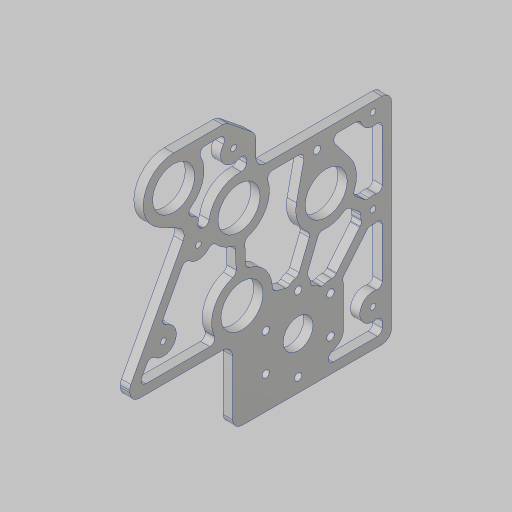
# Autodesk Inventor part: CL4-016
Saved by Autodesk Inventor 2023.5 (Build 275446000, 446)
## iProperties
Created: 2025-02-08
Part Number: CL4-016
Material: Aluminum 6061
Document SubType Name: Modeling
Designer: slick
Density: 2.7 g/cm^3
Appearance: Aluminum - Flat
Author: slick
Autodesk Inventor part; units mm, degrees
ref_plane "YZ Plane" through (0, 0, 0) normal (1, 0, 0) x (0, 1, 0)
ref_plane "XZ Plane" through (0, 0, 0) normal (0, 1, 0) x (-1, 0, 0)
ref_plane "XY Plane" through (0, 0, 0) normal (0, 0, 1) x (1, 0, 0)
sketch "Sketch1" plane through (0, 0, 0) normal (1, 0, 0) x (0, 1, 0)
  line L0 (0, 0) -> (304.8, 0) construction
  line L1 (304.8, 0) -> (304.8, 25.4) construction
  line L2 (304.8, 25.4) -> (0, 25.4) construction
  line L3 (0, 25.4) -> (0, 0) construction
  line L4 (304.8053, 47.8215) -> (292.8807, 25.3947) construction
  line L5 (292.8807, 25.3947) -> (44.6826, 157.364) construction
  line L6 (44.6826, 157.364) -> (56.6072, 179.7908) construction
  line L7 (56.6072, 179.7908) -> (304.8053, 47.8215) construction
  line L8 (50.8, 179.7908) -> (0, 179.7908) construction
  line L9 (0, 179.7908) -> (0, 154.3908) construction
  line L10 (0, 154.3908) -> (50.8, 154.3908) construction
  line L11 (50.8, 154.3908) -> (50.8, 179.7908) construction
  circle A0 centre (320.675, 23.9014) radius 45.3644 construction
  line L12 (0, 0) -> (50.8, 0) construction
  line L13 (50.8, 0) -> (50.8, -25.4) construction
  line L14 (50.8, -25.4) -> (0, -25.4) construction
  line L15 (0, -25.4) -> (0, 0) construction
  line L16 (50.8, -25.4) -> (558.8, -25.4) construction
  point P0 (292.1, 12.7)
  point P1 (304.8, 12.7)
  point P2 (287.6296, 42.5704)
  point P3 (298.843, 36.6081)
  point P4 (0, 167.0908)
  point P5 (0, 12.7)
  dimension "d0" = 25.4
  dimension "d1" = 304.8
  dimension "d2" = 28
  dimension "d3" = 12.7
  dimension "d4" = 12.7
  dimension "d5" = 12.7
  dimension "d6" = 25.4
  dimension "d7" = 281.1018
  dimension "d8" = 4.4704
  dimension "d9" = 29.8704
  dimension "d10" = 50.8
  dimension "d11" = 25.4
  dimension "d12" = 50.8
  dimension "d13" = 25.4
  dimension "d14" = 508
  dimension "d15" = 90.7288
  dimension "d16" = 28.575
  dimension "d17" = 11.2014
  constraints: 34 end point, 8 parallel, 4 horizontal, 4 midpoint, 4 perpendicular, 2 horizontal alignment, 1 centre point, 1 vertical alignment
  measures "d0" distance of L1.end L0.end
  measures "d1" distance of L0.start L0.end
  measures "d2" angle of L2 L5
  measures "d3" distance of point (292.1, 12.7) point (304.8, 12.7)
  measures "d4" distance of point (287.63, 42.57) point (298.843, 36.608)
  measures "d5" distance from line of L7 point (287.63, 42.57)
  measures "d6" distance of L4.start L4.end
  measures "d7" distance of L6.end L4.start
  measures "d8" horizontal distance of point (292.1, 12.7) point (287.63, 42.57)
  measures "d9" vertical distance of point (292.1, 12.7) point (287.63, 42.57)
  measures "d10" distance of L10.end L9.end
  measures "d11" distance of L9.end L8.end
  measures "d12" distance of L13.end L14.end
  measures "d13" distance of L12.end L13.end
  measures "d14" distance of L13.end L16.end
  measures "d15" diameter of A0
  measures "d16" horizontal distance of point (292.1, 12.7) A0.centre
  measures "d17" vertical distance of point (292.1, 12.7) A0.centre
sketch "Sketch2" plane through (0, 0, 0) normal (1, 0, 0) x (0, 1, 0)
  circle A0 centre (320.675, 23.9014) radius 45.3644 construction
  line L0 (50.8, -25.4) -> (558.8, -25.4) construction
  line L1 (50.8, 0) -> (50.8, -25.4) construction
  line L2 (0, 0) -> (50.8, 0) construction
  line L3 (50.8, -25.4) -> (0, -25.4) construction
  line L4 (0, -25.4) -> (0, 0) construction
  line L5 (0, 25.4) -> (0, 0) construction
  line L6 (304.8053, 47.8215) -> (292.8807, 25.3947) construction
  line L7 (304.8, 0) -> (304.8, 25.4) construction
  line L8 (56.6072, 179.7908) -> (304.8053, 47.8215) construction
  line L9 (50.8, 154.3908) -> (50.8, 179.7908) construction
  line L10 (44.6826, 157.364) -> (56.6072, 179.7908) construction
  line L11 (0, 0) -> (304.8, 0) construction
  line L12 (304.8, 25.4) -> (0, 25.4) construction
  line L13 (0, 154.3908) -> (50.8, 154.3908) construction
  line L14 (50.8, 179.7908) -> (0, 179.7908) construction
  line L15 (292.8807, 25.3947) -> (44.6826, 157.364) construction
  line L16 (0, 179.7908) -> (0, 154.3908) construction
  circle A1 centre (34.925, 63.5) radius 30.48 construction
  circle A2 centre (34.925, 63.5) radius 6.35 construction
  circle A3 centre (70.4169, 101.6) radius 45.72 construction
  circle A4 centre (70.4169, 101.6) radius 12.7 construction
  circle A5 centre (128.803, 103.5908) radius 45.72 construction
  circle A6 centre (128.803, 103.5908) radius 12.7 construction
  circle A7 centre (162.718, 148.0019) radius 43.18 construction
  arc A8 (285.6013, 0) -> (341.9337, 60.6371) centre (320.675, 23.9014) ccw construction
  arc A9 (169.8042, 160.2472) -> (152.4976, 138.2191) centre (162.718, 148.0019) ccw construction
  line L17 (169.8042, 160.2472) -> (341.9337, 60.6371) construction
  line L18 (290.0139, -5.4472) -> (152.4976, 138.2191) construction
  circle A10 centre (128.803, 103.5908) radius 14.2875
  circle A11 centre (162.718, 148.0019) radius 14.2875
  circle A12 centre (70.4169, 101.6) radius 14.2875
  circle A13 centre (34.925, 63.5) radius 14.2875 construction
  circle A14 centre (128.803, 103.5908) radius 20.6375 construction
  circle A15 centre (162.718, 148.0019) radius 20.6375 construction
  circle A16 centre (70.4169, 101.6) radius 20.6375 construction
  circle A17 centre (34.925, 63.5) radius 20.6375 construction
  line L19 (185.2061, 97.0299) -> (95.4986, 144.7283) construction
  line L20 (165.1, 12.7) -> (25.4, 12.7) construction
  line L21 (0, 0) -> (190.5, 0)
  line L22 (190.5, 0) -> (190.5, 177.8)
  line L23 (190.5, 177.8) -> (0, 177.8)
  line L24 (0, 177.8) -> (0, 0)
  circle A18 centre (34.925, 63.5) radius 10.16
  circle A19 centre (34.925, 63.5) radius 25.4 construction
  point P0 (0, 12.7)
  point P1 (298.843, 36.6081)
  point P2 (304.8, 12.7)
  point P3 (0, 167.0908)
  point P4 (287.6296, 42.5704)
  point P5 (292.1, 12.7)
  point P6 (140.3524, 120.8791)
  point P7 (95.25, 12.7)
  point P8 (140.3524, 120.8791)
  point P9 (0, 12.7)
  point P10 (95.25, 12.7)
  point P11 (60.325, 63.5)
  point P12 (47.625, 85.497)
  point P13 (22.225, 85.497)
  point P14 (9.525, 63.5)
  point P15 (22.225, 41.503)
  point P16 (47.625, 41.503)
  dimension "d55" = 50.8
  dimension "d18" = 60.96
  dimension "d19" = 34.925
  dimension "d20" = 38.1
  dimension "d21" = 12.7
  dimension "d22" = 91.44
  dimension "d23" = 25.4
  dimension "d24" = 91.44
  dimension "d25" = 25.4
  dimension "d26" = 86.36
  dimension "d27" = 84.8868
  dimension "d28" = 28.2956
  dimension "d29" = 152.3552
  dimension "d30" = 40.4476
  dimension "d31" = 198.8736
  dimension "d32" = 38.1
  dimension "d33" = 50.8
  dimension "d34" = 28.575
  dimension "d35" = 6.35
  dimension "d37" = 12.7
  dimension "d38" = 50.8
  dimension "d39" = 101.6
  dimension "d40" = 139.7
  dimension "d41" = 25.4
  dimension "d42" = 177.8
  dimension "d43" = 190.5
  dimension "d46" = 20.32
  dimension "d58" = 360
  constraints: 18 centre point, 16 end point, 15 coincident, 7 tangent, 6 equal radius, 5 horizontal alignment, 5 point on circle, 3 midpoint, 3 parallel, 2 horizontal, 1 perpendicular, 1 point on line, 9 other
  measures "d18" diameter of A1
  measures "d19" distance from line of A1.centre L5
  measures "d20" distance from line of L12 A1.centre
  measures "d21" diameter of A2
  measures "d22" diameter of A3
  measures "d23" diameter of A4
  measures "d24" diameter of A5
  measures "d25" diameter of A6
  measures "d26" diameter of A7
  measures "d27" diameter of A8
  measures "d28" diameter of A9
  measures "d31" distance of L17.start L17.end
  measures "d32" vertical distance of A2.centre A3.centre
  measures "d33" distance from line of L13 A5.centre
  measures "d34" diameter of A10
  measures "d35" radial gap between concentric circles of A10 A14
  measures "d37" distance between parallel lines of L15 L19
  measures "d38" distance from line of L19.end L10
  measures "d39" distance of L19.start L19.end
  measures "d40" distance of L20.start L20.end
  measures "d41" distance of point (0, 12.7) L20.end
  measures "d42" distance of L21.end L22.end
  measures "d43" distance of L22.end L23.end
  measures "d46" diameter of A18
extrude "Extrusion1" add sketch "Sketch2" along normal blind 6.35
hole "Hole1" at (0, 60.325, 63.5) at (0, 47.625, 41.503) at (0, 22.225, 41.503) at (0, 9.525, 63.5) at (0, 22.225, 85.497) at (0, 47.625, 85.497) direction (1, 0, 0) diameter 5.1054 end through all clearance for "Flat Head Machine Screw (82)" size "#10" standard "Ansi Unified Screw Threads"
sketch "Sketch3" plane through (6.35, 0, 0) normal (1, 0, 0) x (0, 0, -1)
  line L0 (0, 190.5) -> (-177.8, 190.5) projected
  line L1 (0, 190.5) -> (-177.8, 190.5) construction
  line L2 (-177.8, 190.5) -> (-177.8, 0) projected
  line L3 (-177.8, 190.5) -> (-177.8, 0) construction
  line L4 (-177.8, 0) -> (0, 0) projected
  line L5 (-177.8, 0) -> (0, 0) construction
  line L6 (0, 0) -> (0, 190.5) projected
  line L7 (0, 0) -> (0, 190.5) construction
  circle A0 centre (-103.5908, 128.803) radius 14.2875 construction
  circle A1 centre (-103.5908, 128.803) radius 14.2875 construction
  circle A2 centre (-148.0019, 162.718) radius 14.2875 construction
  circle A3 centre (-148.0019, 162.718) radius 14.2875 construction
  circle A4 centre (-101.6, 70.4169) radius 14.2875 construction
  circle A5 centre (-101.6, 70.4169) radius 14.2875 construction
  circle A6 centre (-63.5, 34.925) radius 10.16 construction
  circle A7 centre (-63.5, 34.925) radius 10.16 construction
  line L8 (-25.3947, 292.8807) -> (-157.364, 44.6826) construction
  line L9 (-179.7908, 56.6072) -> (-47.8215, 304.8053) construction
  line L10 (-25.4, 304.8) -> (-25.4, 0) construction
  line L11 (0, 0) -> (0, 304.8) construction
  line L12 (0, 50.8) -> (25.4, 50.8) construction
  line L13 (25.4, 50.8) -> (25.4, 0) construction
  line L14 (25.4, 0) -> (0, 0) construction
  line L15 (-25.4, 0) -> (0, 0) construction
  line L16 (-154.3908, 50.8) -> (-179.7908, 50.8) construction
  line L17 (-157.364, 44.6826) -> (-179.7908, 56.6072) construction
  line L18 (-154.3908, 0) -> (-154.3908, 50.8) construction
  line L19 (-179.7908, 50.8) -> (-179.7908, 0) construction
  line L20 (-179.7908, 0) -> (-154.3908, 0) construction
  line L21 (-47.8215, 304.8053) -> (-25.3947, 292.8807) construction
  line L22 (0, 304.8) -> (-25.4, 304.8) construction
  circle A8 centre (-23.9014, 320.675) radius 45.3644 construction
  line L23 (0, 0) -> (0, 50.8) construction
  line L24 (-107.2912, 165.9075) -> (-154.9895, 76.2) construction
  line L25 (-12.7, 139.7) -> (-12.7, 25.4) construction
  circle A9 centre (-148.0019, 162.718) radius 20.6375 construction
  circle A10 centre (-103.5908, 128.803) radius 20.6375 construction
  circle A11 centre (-101.6, 70.4169) radius 20.6375 construction
  circle A12 centre (-85.497, 22.225) radius 2.5527 construction
  circle A13 centre (-41.503, 22.225) radius 2.5527 construction
  circle A14 centre (-63.5, 60.325) radius 2.5527 construction
  circle A15 centre (-41.503, 47.625) radius 2.5527 construction
  circle A16 centre (-63.5, 9.525) radius 2.5527 construction
  circle A17 centre (-85.497, 47.625) radius 2.5527 construction
  circle A18 centre (-63.5, 34.925) radius 10.16 construction
  circle A19 centre (-101.6, 70.4169) radius 14.2875 construction
  circle A20 centre (-148.0019, 162.718) radius 14.2875 construction
  circle A21 centre (-103.5908, 128.803) radius 14.2875 construction
  line L26 (0, 190.5) -> (0, 0) construction
  line L27 (0, 0) -> (-177.8, 0) construction
  line L28 (-177.8, 0) -> (-177.8, 190.5) construction
  line L29 (-177.8, 190.5) -> (0, 190.5) construction
  circle A22 centre (-63.5, 60.325) radius 8.9027 construction
  circle A23 centre (-85.497, 47.625) radius 8.9027 construction
  circle A24 centre (-85.497, 22.225) radius 8.9027 construction
  circle A25 centre (-63.5, 9.525) radius 2.5527 construction
  circle A26 centre (-63.5, 9.525) radius 8.9027 construction
  circle A27 centre (-41.503, 22.225) radius 2.5527 construction
  circle A28 centre (-41.503, 22.225) radius 8.9027 construction
  circle A29 centre (-41.503, 47.625) radius 2.5527 construction
  circle A30 centre (-41.503, 47.625) radius 8.9027 construction
  line L30 (-148.0019, 183.3555) -> (-112.3976, 183.3555)
  line L31 (0, 146.05) -> (-92.2574, 146.05)
  line L32 (-92.2574, 146.05) -> (-92.2574, 167.1302)
  line L33 (-112.3976, 183.3555) -> (-92.2574, 167.1302)
  line L34 (-157.6907, 144.4962) -> (-138.4882, 134.2861)
  line L35 (-138.4882, 134.2861) -> (-177.8, 60.3514)
  line L36 (-154.3908, 50.8) -> (-108.0097, 50.8)
  line L37 (-108.0097, 50.8) -> (-108.0097, 0)
  line L38 (-108.0097, 0) -> (0, 0)
  line L39 (0, 0) -> (0, 146.05)
  arc A31 (-148.0019, 183.3555) -> (-157.6907, 144.4962) centre (-148.0019, 162.718) ccw
  line L40 (-177.8, 60.3514) -> (-177.8, 50.8)
  line L41 (-154.3908, 50.8) -> (-177.8, 50.8)
  circle A32 centre (-103.5908, 128.803) radius 7.62
  point P0 (-12.7, 0)
  point P1 (-167.0908, 0)
  point P2 (-12.7, 304.8)
  point P3 (-36.6081, 298.843)
  point P4 (-42.5704, 287.6296)
  point P5 (-12.7, 292.1)
  point P6 (-131.1404, 121.0537)
  point P7 (-12.7, 82.55)
  point P8 (-12.7, 25.4)
  point P9 (-131.1404, 121.0537)
  point P10 (-12.7, 82.55)
  point P11 (-108.0097, 0)
  dimension "d47" = 12.7
  dimension "d48" = 25.4
  dimension "d49" = 101.6
  dimension "d50" = 25.4
  dimension "d51" = 114.3
  dimension "d52" = 6.35
  dimension "d53" = 6.35
  dimension "d54" = 6.35
  dimension "d67" = 6.35
  dimension "d68" = 6.35
  dimension "d90" = 15.24
  constraints: 28 end point, 11 coincident, 9 centre point, 9 point on line, 5 equal radius, 5 perpendicular, 4 point on circle, 3 vertical alignment, 2 collinear, 2 midpoint, 2 tangent, 2 vertical, 1 horizontal, 1 parallel, 6 other
  measures "d47" distance between parallel lines of L9 L24
  measures "d48" distance from line of L16 L24.end
  measures "d49" distance of L24.start L24.end
  measures "d50" distance from line of L15 point (-12.7, 25.4)
  measures "d51" distance of L25.start L25.end
  measures "d52" radial gap between concentric circles of A2 A9
  measures "d67" radial gap between concentric circles of A14 A22
  measures "d68" vertical distance of L31.start L25.start
  measures "d90" diameter of A32
extrude "Extrusion2" cut sketch "Sketch3" against normal through all contours L6 L31 L32 L33 L30 A31 L34 L35 L2 L0 | L41 L36 L37 L4 L2
hole "Hole2" at (6.35, 304.8, 12.7) at (6.35, 320.675, 23.9014) at (6.35, 298.843, 36.6081) at (6.35, 287.6296, 42.5704) at (6.35, 292.1, 12.7) at (6.35, 76.2, 154.9895) at (6.35, 121.0537, 131.1404) at (6.35, 165.9075, 107.2912) at (6.35, 139.7, 12.7) at (6.35, 82.55, 12.7) at (6.35, 25.4, 12.7) direction (-1, 0, 0) diameter 3.9624 end through all thread size "10-32 UNF" class "2B" standard "ANSI Unified Screw Threads"
sketch "Sketch4" plane through (6.35, 0, 0) normal (1, 0, 0) x (0, 0, -1)
  circle A0 centre (-12.7, 82.55) radius 1.9812 construction
  circle A1 centre (-107.2912, 165.9075) radius 1.9812 construction
  circle A2 centre (-154.9895, 76.2) radius 1.9812 construction
  circle A3 centre (-131.1404, 121.0537) radius 1.9812 construction
  circle A4 centre (-12.7, 139.7) radius 1.9812 construction
  circle A5 centre (-12.7, 25.4) radius 1.9812 construction
  line L0 (-177.8, 60.3514) -> (-138.4882, 134.2861) construction
  line L1 (-138.4882, 134.2861) -> (-157.6907, 144.4962) construction
  arc A6 (-148.0019, 183.3555) -> (-157.6907, 144.4962) centre (-148.0019, 162.718) ccw construction
  line L2 (-148.0019, 183.3555) -> (-112.3976, 183.3555) construction
  line L3 (-112.3976, 183.3555) -> (-92.2574, 167.1302) construction
  line L4 (-92.2574, 167.1302) -> (-92.2574, 146.05) construction
  line L5 (-92.2574, 146.05) -> (0, 146.05) construction
  line L6 (0, 146.05) -> (0, 0) construction
  line L7 (0, 0) -> (-108.0097, 0) construction
  line L8 (-108.0097, 0) -> (-108.0097, 50.8) construction
  line L9 (-108.0097, 50.8) -> (-177.8, 50.8) construction
  line L10 (-177.8, 50.8) -> (-177.8, 60.3514) construction
  circle A7 centre (-85.497, 22.225) radius 2.5527 construction
  circle A8 centre (-41.503, 22.225) radius 2.5527 construction
  circle A9 centre (-63.5, 60.325) radius 2.5527 construction
  circle A10 centre (-41.503, 47.625) radius 2.5527 construction
  circle A11 centre (-63.5, 9.525) radius 2.5527 construction
  circle A12 centre (-85.497, 47.625) radius 2.5527 construction
  circle A13 centre (-63.5, 34.925) radius 10.16 construction
  circle A14 centre (-101.6, 70.4169) radius 14.2875 construction
  circle A15 centre (-148.0019, 162.718) radius 14.2875 construction
  circle A16 centre (-103.5908, 128.803) radius 14.2875 construction
  line L11 (-6.35, 139.7) -> (-98.6074, 139.7) construction
  line L12 (-98.6074, 139.7) -> (-98.6074, 164.0916) construction
  line L13 (-98.6074, 164.0916) -> (-114.6372, 177.0055) construction
  line L14 (-114.6372, 177.0055) -> (-148.0019, 177.0055) construction
  arc A17 (-148.0019, 177.0055) -> (-154.7095, 150.1029) centre (-148.0019, 162.718) ccw construction
  line L15 (-154.7095, 150.1029) -> (-129.9004, 136.9116) construction
  line L16 (-129.9004, 136.9116) -> (-171.45, 58.7682) construction
  line L17 (-171.45, 58.7682) -> (-171.45, 57.15) construction
  line L18 (-171.45, 57.15) -> (-101.6597, 57.15) construction
  line L19 (-101.6597, 57.15) -> (-101.6597, 6.35) construction
  line L20 (-101.6597, 6.35) -> (-6.35, 6.35) construction
  line L21 (-6.35, 6.35) -> (-6.35, 139.7) construction
  circle A18 centre (-103.5908, 128.803) radius 20.6375 construction
  circle A19 centre (-63.5, 60.325) radius 8.9027 construction
  circle A20 centre (-154.9895, 76.2) radius 1.9812 construction
  circle A21 centre (-154.9895, 76.2) radius 8.9027 construction
  circle A22 centre (-131.1404, 121.0537) radius 1.9812 construction
  circle A23 centre (-131.1404, 121.0537) radius 8.9027 construction
  circle A24 centre (-107.2912, 165.9075) radius 1.9812 construction
  circle A25 centre (-107.2912, 165.9075) radius 8.9027 construction
  circle A26 centre (-85.497, 47.625) radius 2.5527 construction
  circle A27 centre (-85.497, 47.625) radius 8.9027 construction
  circle A28 centre (-41.503, 47.625) radius 2.5527 construction
  circle A29 centre (-41.503, 47.625) radius 8.9027 construction
  circle A30 centre (-12.7, 82.55) radius 1.9812 construction
  circle A31 centre (-12.7, 82.55) radius 8.9027 construction
  circle A32 centre (-12.7, 139.7) radius 1.9812 construction
  circle A33 centre (-12.7, 139.7) radius 8.9027 construction
  circle A34 centre (-12.7, 25.4) radius 1.9812 construction
  circle A35 centre (-12.7, 25.4) radius 8.9027 construction
  circle A36 centre (-41.503, 22.225) radius 2.5527 construction
  circle A37 centre (-41.503, 22.225) radius 8.9027 construction
  circle A38 centre (-85.497, 22.225) radius 8.9027 construction
  circle A39 centre (-101.6, 70.4169) radius 20.6375 construction
  circle A40 centre (-148.0019, 162.718) radius 20.6375 construction
  line L22 (-103.5908, 128.803) -> (-101.6, 70.4169) construction
  line L23 (-101.6, 70.4169) -> (-12.7, 139.7) construction
  line L24 (-41.503, 47.625) -> (-12.7, 82.55) construction
  line L25 (-14.6517, 142.2043) -> (-98.6391, 76.7498) construction
  line L26 (-98.6391, 76.7498) -> (-100.4177, 128.9112) construction
  line L27 (-10.7483, 137.1957) -> (-104.5609, 64.084) construction
  line L28 (-104.5609, 64.084) -> (-106.764, 128.6948) construction
  line L29 (-39.0535, 45.6049) -> (-10.2505, 80.5299) construction
  line L30 (-141.5606, 143.1115) -> (-129.9004, 136.9116)
  line L31 (-129.9004, 136.9116) -> (-133.8176, 129.5443)
  line L32 (-133.1099, 177.0055) -> (-114.6372, 177.0055)
  line L33 (-114.6372, 177.0055) -> (-110.9409, 174.0277)
  line L34 (-98.6074, 164.0916) -> (-98.6074, 148.8297)
  line L35 (-86.0648, 139.7) -> (-21.6027, 139.7)
  line L36 (-21.212, 137.0916) -> (-87.4675, 85.4562)
  line L37 (-99.1218, 90.9051) -> (-99.7228, 108.5312)
  line L38 (-83.5642, 80.4476) -> (-17.3086, 132.083)
  line L39 (-6.35, 133.4602) -> (-6.35, 88.7898)
  line L40 (-6.35, 76.3102) -> (-6.35, 31.6398)
  line L41 (-6.35, 19.1602) -> (-6.35, 6.35)
  circle A41 centre (-63.5, 9.525) radius 2.5527 construction
  circle A42 centre (-63.5, 9.525) radius 8.9027 construction
  line L42 (-6.35, 6.35) -> (-55.1827, 6.35)
  line L43 (-55.1827, 6.35) -> (-37.8666, 14.0988)
  line L44 (-32.6003, 22.225) -> (-32.6003, 47.625)
  line L45 (-33.7616, 52.0216) -> (-15.5424, 74.1133)
  line L46 (-38.5476, 56.1987) -> (-20.4413, 78.1534)
  line L47 (-38.5476, 56.1987) -> (-59.0486, 68.035)
  line L48 (-67.9513, 68.035) -> (-89.9484, 55.335)
  line L49 (-106.0691, 108.3148) -> (-105.4681, 90.6887)
  line L50 (-117.4081, 57.15) -> (-171.45, 57.15)
  line L51 (-171.45, 57.15) -> (-171.45, 58.7682)
  line L52 (-171.45, 58.7682) -> (-163.5257, 73.6717)
  line L53 (-157.6668, 84.6906) -> (-139.6765, 118.5254)
  arc A43 (-139.6765, 118.5254) -> (-122.2917, 120.0745) centre (-131.1404, 121.0537) ccw
  arc A44 (-122.2917, 120.0745) -> (-106.0691, 108.3148) centre (-103.5908, 128.803) ccw
  arc A45 (-99.7228, 108.5312) -> (-86.0648, 139.7) centre (-103.5908, 128.803) ccw
  arc A46 (-21.6027, 139.7) -> (-21.212, 137.0916) centre (-12.7, 139.7) ccw
  arc A47 (-17.3086, 132.083) -> (-6.35, 133.4602) centre (-12.7, 139.7) ccw
  arc A48 (-6.35, 88.7898) -> (-20.4413, 78.1534) centre (-12.7, 82.55) ccw
  arc A49 (-15.5424, 74.1133) -> (-6.35, 76.3102) centre (-12.7, 82.55) ccw
  arc A50 (-6.35, 31.6398) -> (-6.35, 19.1602) centre (-12.7, 25.4) ccw
  arc A51 (-37.8666, 14.0988) -> (-32.6003, 22.225) centre (-41.503, 22.225) ccw
  arc A52 (-32.6003, 47.625) -> (-33.7616, 52.0216) centre (-41.503, 47.625) ccw
  arc A53 (-59.0486, 68.035) -> (-67.9513, 68.035) centre (-63.5, 60.325) ccw
  arc A54 (-84.9532, 58.219) -> (-83.5642, 80.4476) centre (-101.6, 70.4169) ccw
  arc A55 (-105.4681, 90.6887) -> (-117.4081, 57.15) centre (-101.6, 70.4169) ccw
  arc A56 (-163.5257, 73.6717) -> (-157.6668, 84.6906) centre (-154.9895, 76.2) ccw
  arc A57 (-141.5606, 143.1115) -> (-133.1099, 177.0055) centre (-148.0019, 162.718) ccw
  arc A58 (-110.9409, 174.0277) -> (-98.6074, 163.9453) centre (-107.2912, 165.9075) ccw
  arc A59 (-98.6074, 148.8297) -> (-124.0997, 126.5024) centre (-103.5908, 128.803) ccw
  arc A60 (-124.0997, 126.5024) -> (-133.8176, 129.5443) centre (-131.1404, 121.0537) ccw
  line L54 (-43.9524, 49.6451) -> (-38.6605, 56.0617) construction
  line L55 (-38.5476, 56.1987) -> (-15.1495, 84.5701) construction
  arc A61 (-87.4675, 85.4562) -> (-99.1218, 90.9051) centre (-101.6, 70.4169) ccw
  dimension "d78" = 6.35
  dimension "d79" = 6.35
  dimension "d80" = 6.35
  dimension "d81" = 3.175
  dimension "d82" = 3.175
  dimension "d84" = 3.175
  dimension "d85" = 3.175
  constraints: 90 end point, 79 point on circle, 33 centre point, 30 coincident, 30 point on line, 10 equal radius, 5 tangent, 4 collinear, 3 parallel, 2 perpendicular, 1 concentric, 1 vertical, 23 other
  measures "d78" distance between parallel lines of L5 L11
  measures "d79" radial gap between concentric circles of A16 A18
  measures "d80" radial gap between concentric circles of A9 A19
  measures "d81" distance between parallel lines of L23 L25
  measures "d82" distance between parallel lines of L23 L27
  measures "d84" distance between parallel lines of L24 L29
  measures "d85" distance between parallel lines of L24 L46
extrude "Extrusion3" cut sketch "Sketch4" against normal through all contours A57 L32 L33 A58 L34 A59 A60 L31 L30 | L40 A50 L41 L42 L43 A51 L44 A52 L45 A49 | L49 A55 L50 L51 L52 A56 L53 A43 A44
fillet "Fillet1" radius 3.302 25 edges at (3.175, 57.15, 117.4081) (3.175, 90.6887, 105.4681) (3.175, 108.3148, 106.0691) (3.175, 120.0745, 122.2917) (3.175, 118.5254, 139.6765) (3.175, 84.6906, 157.6668) (3.175, 73.6717, 163.5257) (3.175, 58.7682, 171.45) (3.175, 57.15, 171.45) (3.175, 6.35, 6.35) (3.175, 19.1602, 6.35) (3.175, 31.6398, 6.35) (3.175, 76.3102, 6.35) (3.175, 74.1133, 15.5424) (3.175, 52.0216, 33.7616) (3.175, 6.35, 55.1827) (3.175, 148.8297, 98.6074) (3.175, 163.9453, 98.6074) (3.175, 174.0277, 110.9409) (3.175, 177.0055, 114.6372) (3.175, 177.0055, 133.1099) (3.175, 143.1115, 141.5606) (3.175, 136.9116, 129.9004) (3.175, 129.5443, 133.8176) (3.175, 126.5024, 124.0997)
fillet "Fillet2" radius 6.604 10 edges at (3.175, 50.8, 108.0097) (3.175, 183.3555, 112.3976) (3.175, 167.1302, 92.2574) (3.175, 146.05, 92.2574) (3.175, 134.2861, 138.4882) (3.175, 60.3514, 177.8) (3.175, 50.8, 177.8) (3.175, 0, 108.0097) (3.175, 0, 0) (3.175, 146.05, 0)
sketch "Sketch5" plane through (6.35, 0, 0) normal (1, 0, 0) x (0, 0, -1)
  circle A0 centre (-44.45, 107.95) radius 14.2875
  line L0 (0, 6.604) -> (0, 139.446) construction
  line L1 (-6.604, 146.05) -> (-85.6534, 146.05) construction
  point P0 (0, 0)
  dimension "d91" = 28.575
  dimension "d92" = 44.45
  dimension "d93" = 38.1
  constraints: 1 centre point
  measures "d91" diameter of A0
  measures "d92" distance from line of L0 A0.centre
  measures "d93" distance from line of A0.centre L1
extrude "Extrusion4" cut sketch "Sketch5" against normal through all
sketch "Sketch6" plane through (6.35, 0, 0) normal (1, 0, 0) x (0, 0, -1)
  line L0 (-6.604, 146.05) -> (-85.6534, 146.05) construction
  line L1 (0, 6.604) -> (0, 139.446) construction
  point P0 (0, 0)
  point P1 (-50.8, 136.525)
  dimension "d96" = 9.525
  dimension "d97" = 50.8
  measures "d96" distance from line of L0 point (-50.8, 136.525)
  measures "d97" distance from line of L1 point (-50.8, 136.525)
hole "Hole3" at (6.35, 136.525, 50.8) direction (-1, 0, 0) diameter 5.1054 end through all clearance for "Flat Head Machine Screw (82)" size "#10" standard "Ansi Unified Screw Threads"
sketch "Sketch7" plane through (6.35, 0, 0) normal (1, 0, 0) x (0, 0, -1)
  circle A0 centre (-50.8, 136.525) radius 2.5527 construction
  circle A1 centre (-44.45, 107.95) radius 14.2875 construction
  arc A2 (0, 139.446) -> (-6.604, 146.05) centre (-6.604, 139.446) ccw construction
  line L0 (-6.604, 146.05) -> (-85.6534, 146.05) construction
  arc A3 (-92.2574, 152.654) -> (-85.6534, 146.05) centre (-85.6534, 152.654) ccw construction
  line L1 (-92.2574, 152.654) -> (-92.2574, 163.97) construction
  arc A4 (-92.2574, 163.97) -> (-94.7183, 169.1128) centre (-98.8614, 163.97) ccw construction
  line L2 (-94.7183, 169.1128) -> (-110.5837, 181.8942) construction
  arc A5 (-110.5837, 181.8942) -> (-114.7268, 183.3555) centre (-114.7268, 176.7515) ccw construction
  line L3 (-114.7268, 183.3555) -> (-148.0019, 183.3555) construction
  arc A6 (-148.0019, 183.3555) -> (-157.6907, 144.4962) centre (-148.0019, 162.718) ccw construction
  line L4 (-157.6907, 144.4962) -> (-144.3192, 137.3865) construction
  arc A7 (-141.5886, 128.4551) -> (-144.3192, 137.3865) centre (-147.4196, 131.5555) ccw construction
  line L5 (-141.5886, 128.4551) -> (-177.027, 61.8052) construction
  arc A8 (-177.027, 61.8052) -> (-177.8, 58.7048) centre (-171.196, 58.7048) ccw construction
  line L6 (-177.8, 58.7048) -> (-177.8, 57.404) construction
  arc A9 (-177.8, 57.404) -> (-171.196, 50.8) centre (-171.196, 57.404) ccw construction
  line L7 (-171.196, 50.8) -> (-114.6137, 50.8) construction
  arc A10 (-108.0097, 44.196) -> (-114.6137, 50.8) centre (-114.6137, 44.196) ccw construction
  line L8 (-108.0097, 44.196) -> (-108.0097, 6.604) construction
  arc A11 (-108.0097, 6.604) -> (-101.4057, 0) centre (-101.4057, 6.604) ccw construction
  line L9 (-101.4057, 0) -> (-6.604, 0) construction
  arc A12 (-6.604, 0) -> (0, 6.604) centre (-6.604, 6.604) ccw construction
  line L10 (0, 6.604) -> (0, 139.446) construction
  arc A13 (-131.3354, 134.2354) -> (-132.8159, 138.4618) centre (-134.3661, 135.5463) ccw construction
  line L11 (-132.8159, 138.4618) -> (-135.9291, 140.1172) construction
  arc A14 (-136.2579, 145.7479) -> (-135.9291, 140.1172) centre (-134.3789, 143.0327) ccw construction
  arc A15 (-136.2579, 145.7479) -> (-129.6656, 172.1883) centre (-148.0019, 162.718) ccw construction
  arc A16 (-126.7318, 177.0055) -> (-129.6656, 172.1883) centre (-126.7318, 173.7035) ccw construction
  line L12 (-126.7318, 177.0055) -> (-116.6814, 177.0055) construction
  arc A17 (-114.1409, 171.5943) -> (-116.6814, 177.0055) centre (-116.6814, 173.7035) ccw construction
  arc A18 (-114.1409, 171.5943) -> (-103.3655, 157.9171) centre (-107.2912, 165.9075) ccw construction
  arc A19 (-98.6074, 154.9534) -> (-103.3655, 157.9171) centre (-101.9094, 154.9534) ccw construction
  line L13 (-98.6074, 154.9534) -> (-98.6074, 152.6833) construction
  arc A20 (-102.1414, 149.3895) -> (-98.6074, 152.6833) centre (-101.9094, 152.6833) ccw construction
  arc A21 (-102.1414, 149.3895) -> (-123.9652, 132.0878) centre (-103.5908, 128.803) ccw construction
  arc A22 (-128.2844, 129.4859) -> (-123.9652, 132.0878) centre (-127.2251, 132.6134) ccw construction
  arc A23 (-128.2844, 129.4859) -> (-129.072, 129.7128) centre (-131.1404, 121.0537) ccw construction
  arc A24 (-131.3354, 134.2354) -> (-129.072, 129.7128) centre (-128.3048, 132.9245) ccw construction
  arc A25 (-32.6003, 47.625) -> (-33.0571, 50.4402) centre (-41.503, 47.625) ccw construction
  arc A26 (-32.472, 53.5853) -> (-33.0571, 50.4402) centre (-29.9245, 51.4844) ccw construction
  line L14 (-32.472, 53.5853) -> (-16.8321, 72.5495) construction
  arc A27 (-13.8559, 73.7227) -> (-16.8321, 72.5495) centre (-14.2846, 70.4486) ccw construction
  arc A28 (-13.8559, 73.7227) -> (-10.4766, 73.9294) centre (-12.7, 82.55) ccw construction
  arc A29 (-6.35, 70.732) -> (-10.4766, 73.9294) centre (-9.652, 70.732) ccw construction
  line L15 (-6.35, 70.732) -> (-6.35, 37.218) construction
  arc A30 (-10.4766, 34.0206) -> (-6.35, 37.218) centre (-9.652, 37.218) ccw construction
  arc A31 (-10.4766, 34.0206) -> (-10.4766, 16.7794) centre (-12.7, 25.4) ccw construction
  arc A32 (-6.35, 13.582) -> (-10.4766, 16.7794) centre (-9.652, 13.582) ccw construction
  line L16 (-6.35, 13.582) -> (-6.35, 9.652) construction
  arc A33 (-9.652, 6.35) -> (-6.35, 9.652) centre (-9.652, 9.652) ccw construction
  line L17 (-9.652, 6.35) -> (-39.7198, 6.35) construction
  arc A34 (-41.0685, 12.666) -> (-39.7198, 6.35) centre (-39.7198, 9.652) ccw construction
  line L18 (-41.0685, 12.666) -> (-37.8666, 14.0988) construction
  arc A35 (-37.8666, 14.0988) -> (-32.6003, 22.225) centre (-41.503, 22.225) ccw construction
  line L19 (-32.6003, 22.225) -> (-32.6003, 47.625) construction
  arc A36 (-169.7304, 62.0022) -> (-166.8149, 57.15) centre (-166.8149, 60.452) ccw construction
  line L20 (-169.7304, 62.0022) -> (-166.1444, 68.7465) construction
  arc A37 (-160.9997, 69.6323) -> (-166.1444, 68.7465) centre (-163.2289, 67.1963) ccw construction
  arc A38 (-160.9997, 69.6323) -> (-152.9055, 84.8553) centre (-154.9895, 76.2) ccw construction
  arc A39 (-155.048, 89.6158) -> (-152.9055, 84.8553) centre (-152.1325, 88.0656) ccw construction
  line L21 (-155.048, 89.6158) -> (-142.2953, 113.6002) construction
  arc A40 (-137.1506, 114.486) -> (-142.2953, 113.6002) centre (-139.3798, 112.05) ccw construction
  arc A41 (-137.1506, 114.486) -> (-124.3073, 115.3469) centre (-131.1404, 121.0537) ccw construction
  arc A42 (-119.2651, 115.3782) -> (-124.3073, 115.3469) centre (-121.773, 113.2302) ccw construction
  arc A43 (-119.2651, 115.3782) -> (-108.4942, 108.7564) centre (-103.5908, 128.803) ccw construction
  arc A44 (-105.9786, 105.6615) -> (-108.4942, 108.7564) centre (-109.2787, 105.549) ccw construction
  line L22 (-105.9786, 105.6615) -> (-105.5585, 93.342) construction
  arc A45 (-107.8574, 90.0829) -> (-105.5585, 93.342) centre (-108.8586, 93.2294) ccw construction
  arc A46 (-107.8574, 90.0829) -> (-120.3646, 61.8265) centre (-101.6, 70.4169) ccw construction
  arc A47 (-123.367, 57.15) -> (-120.3646, 61.8265) centre (-123.367, 60.452) ccw construction
  line L23 (-123.367, 57.15) -> (-166.8149, 57.15) construction
  circle A48 centre (-12.7, 82.55) radius 1.9812 construction
  circle A49 centre (-107.2912, 165.9075) radius 1.9812 construction
  circle A50 centre (-154.9895, 76.2) radius 1.9812 construction
  circle A51 centre (-131.1404, 121.0537) radius 1.9812 construction
  circle A52 centre (-12.7, 139.7) radius 1.9812 construction
  circle A53 centre (-12.7, 25.4) radius 1.9812 construction
  circle A54 centre (-63.5, 34.925) radius 10.16 construction
  circle A55 centre (-101.6, 70.4169) radius 14.2875 construction
  circle A56 centre (-148.0019, 162.718) radius 14.2875 construction
  circle A57 centre (-103.5908, 128.803) radius 14.2875 construction
  circle A58 centre (-85.497, 47.625) radius 2.5527 construction
  circle A59 centre (-63.5, 9.525) radius 2.5527 construction
  circle A60 centre (-41.503, 47.625) radius 2.5527 construction
  circle A61 centre (-63.5, 60.325) radius 2.5527 construction
  circle A62 centre (-41.503, 22.225) radius 2.5527 construction
  circle A63 centre (-85.497, 22.225) radius 2.5527 construction
  line L24 (-85.6534, 139.7) -> (-6.604, 139.7) construction
  arc A64 (-6.35, 139.446) -> (-6.604, 139.7) centre (-6.604, 139.446) ccw construction
  line L25 (-6.35, 139.446) -> (-6.35, 6.604) construction
  arc A65 (-6.604, 6.35) -> (-6.35, 6.604) centre (-6.604, 6.604) ccw construction
  line L26 (-6.604, 6.35) -> (-101.4057, 6.35) construction
  arc A66 (-101.6597, 6.604) -> (-101.4057, 6.35) centre (-101.4057, 6.604) ccw construction
  line L27 (-101.6597, 6.604) -> (-101.6597, 44.196) construction
  arc A67 (-101.6597, 44.196) -> (-114.6137, 57.15) centre (-114.6137, 44.196) ccw construction
  line L28 (-114.6137, 57.15) -> (-171.196, 57.15) construction
  arc A68 (-171.45, 57.404) -> (-171.196, 57.15) centre (-171.196, 57.404) ccw construction
  line L29 (-171.45, 57.404) -> (-171.45, 58.7048) construction
  arc A69 (-171.4203, 58.8241) -> (-171.45, 58.7048) centre (-171.196, 58.7048) ccw construction
  line L30 (-171.4203, 58.8241) -> (-135.9819, 125.4739) construction
  arc A70 (-135.9819, 125.4739) -> (-141.3381, 142.9932) centre (-147.4196, 131.5555) ccw construction
  line L31 (-141.3381, 142.9932) -> (-154.7095, 150.1029) construction
  arc A71 (-148.0019, 177.0055) -> (-154.7095, 150.1029) centre (-148.0019, 162.718) ccw construction
  line L32 (-148.0019, 177.0055) -> (-114.7268, 177.0055) construction
  arc A72 (-114.5675, 176.9493) -> (-114.7268, 177.0055) centre (-114.7268, 176.7515) ccw construction
  line L33 (-114.5675, 176.9493) -> (-98.7021, 164.1678) construction
  arc A73 (-98.6074, 163.97) -> (-98.7021, 164.1678) centre (-98.8614, 163.97) ccw construction
  line L34 (-98.6074, 163.97) -> (-98.6074, 152.654) construction
  arc A74 (-98.6074, 152.654) -> (-85.6534, 139.7) centre (-85.6534, 152.654) ccw construction
  circle A75 centre (-44.45, 107.95) radius 20.6375 construction
  circle A76 centre (-12.7, 82.55) radius 8.3312 construction
  circle A77 centre (-63.5, 60.325) radius 8.3312 construction
  circle A78 centre (-50.8, 136.525) radius 2.5527 construction
  circle A79 centre (-50.8, 136.525) radius 8.3312 construction
  circle A80 centre (-103.5908, 128.803) radius 20.6375 construction
  circle A81 centre (-101.6, 70.4169) radius 20.6375 construction
  circle A82 centre (-12.7, 82.55) radius 1.9812 construction
  line L35 (-12.7, 82.55) -> (-44.45, 107.95) construction
  line L36 (-44.45, 107.95) -> (-63.5, 60.325) construction
  line L37 (-63.5, 60.325) -> (-101.6, 70.4169) construction
  circle A83 centre (-103.5908, 128.803) radius 14.2875 construction
  line L38 (-101.6, 70.4169) -> (-103.5908, 128.803) construction
  line L39 (-100.4177, 128.9112) -> (-98.5072, 72.8822) construction
  line L40 (-98.5072, 72.8822) -> (-65.404, 64.1138) construction
  line L41 (-65.404, 64.1138) -> (-45.8085, 113.1028) construction
  line L42 (-45.8085, 113.1028) -> (-10.7166, 85.0293) construction
  line L43 (-106.764, 128.6948) -> (-104.6928, 67.9516) construction
  line L44 (-104.6928, 67.9516) -> (-61.596, 56.5362) construction
  line L45 (-61.596, 56.5362) -> (-43.0915, 102.7972) construction
  line L46 (-43.0915, 102.7972) -> (-14.6834, 80.0707) construction
  circle A84 centre (-12.7, 139.7) radius 1.9812 construction
  circle A85 centre (-12.7, 139.7) radius 8.3312 construction
  line L47 (-99.7228, 108.5312) -> (-99.1218, 90.9051)
  line L48 (-81.075, 68.2648) -> (-70.1328, 65.3664)
  line L49 (-63.5873, 68.6557) -> (-54.9712, 90.1958)
  line L50 (-30.5101, 92.7321) -> (-20.698, 84.8824)
  line L51 (-16.7312, 89.841) -> (-26.5433, 97.6906)
  line L52 (-49.0754, 87.8375) -> (-57.6915, 66.2974)
  line L53 (-71.7587, 59.2281) -> (-83.1444, 62.2439)
  line L54 (-85.6534, 139.7) -> (-58.5025, 139.7)
  line L55 (-43.0975, 139.7) -> (-21.0312, 139.7)
  line L56 (-6.35, 134.3068) -> (-6.35, 87.9432)
  line L57 (-21.731, 76.5897) -> (-37.3709, 57.6255) construction
  arc A86 (-37.3709, 57.6255) -> (-39.0812, 48.4322) centre (-29.9245, 51.4844) ccw construction
  arc A87 (-38.9503, 47.625) -> (-39.0812, 48.4322) centre (-41.503, 47.625) ccw construction
  line L58 (-38.9503, 47.625) -> (-38.9503, 22.225) construction
  arc A88 (-40.4603, 19.895) -> (-38.9503, 22.225) centre (-41.503, 22.225) ccw construction
  line L59 (-40.4603, 19.895) -> (-43.6622, 18.4621) construction
  arc A89 (-43.6622, 18.4621) -> (-39.7198, 0) centre (-39.7198, 9.652) ccw construction
  line L60 (-39.7198, 0) -> (-9.652, 0) construction
  arc A90 (-9.652, 0) -> (0, 9.652) centre (-9.652, 9.652) ccw construction
  line L61 (0, 9.652) -> (0, 13.582) construction
  arc A91 (0, 13.582) -> (-12.0625, 22.9282) centre (-9.652, 13.582) ccw construction
  arc A92 (-12.0625, 27.8718) -> (-12.0625, 22.9282) centre (-12.7, 25.4) ccw construction
  arc A93 (-12.0625, 27.8718) -> (0, 37.218) centre (-9.652, 37.218) ccw construction
  line L62 (0, 37.218) -> (0, 70.732) construction
  arc A94 (0, 70.732) -> (-12.0625, 80.0782) centre (-9.652, 70.732) ccw construction
  arc A95 (-13.0314, 80.0189) -> (-12.0625, 80.0782) centre (-12.7, 82.55) ccw construction
  arc A96 (-13.0314, 80.0189) -> (-21.731, 76.5897) centre (-14.2846, 70.4486) ccw construction
  circle A97 centre (-41.503, 47.625) radius 2.5527 construction
  circle A98 centre (-41.503, 47.625) radius 8.3312 construction
  line L63 (-63.5, 60.325) -> (-41.503, 47.625) construction
  line L64 (-39.9155, 50.3746) -> (-62.2785, 63.2859) construction
  line L65 (-62.2785, 63.2859) -> (-98.5072, 72.8822) construction
  line L66 (-98.5072, 72.8822) -> (-100.4177, 128.9112) construction
  line L67 (-55.242, 59.2234) -> (-46.586, 54.2259)
  line L68 (-37.3709, 57.6255) -> (-21.731, 76.5897)
  arc A99 (-58.5025, 139.7) -> (-58.939, 138.3043) centre (-50.8, 136.525) ccw
  arc A100 (-64.6113, 112.3576) -> (-54.9712, 90.1958) centre (-44.45, 107.95) ccw
  arc A101 (-26.5433, 97.6906) -> (-28.0529, 120.4817) centre (-44.45, 107.95) ccw
  arc A102 (-21.0312, 139.7) -> (-6.35, 134.3068) centre (-12.7, 139.7) ccw
  arc A103 (-6.35, 87.9432) -> (-16.7312, 89.841) centre (-12.7, 82.55) ccw
  arc A104 (-20.698, 84.8824) -> (-19.8754, 78.3165) centre (-12.7, 82.55) ccw
  arc A105 (-19.8754, 78.3165) -> (-21.731, 76.5897) centre (-14.2846, 70.4486) ccw
  arc A106 (-37.3709, 57.6255) -> (-38.7129, 55.4751) centre (-29.9245, 51.4844) ccw
  arc A107 (-38.7129, 55.4751) -> (-46.586, 54.2259) centre (-41.503, 47.625) ccw
  arc A108 (-55.242, 59.2234) -> (-57.6915, 66.2974) centre (-63.5, 60.325) ccw
  arc A109 (-63.5873, 68.6557) -> (-70.1328, 65.3664) centre (-63.5, 60.325) ccw
  arc A110 (-81.075, 68.2648) -> (-99.1218, 90.9051) centre (-101.6, 70.4169) ccw
  line L69 (-58.939, 138.3043) -> (-64.6113, 112.3576)
  line L70 (-44.1806, 141.5839) -> (-28.0529, 120.4817)
  arc A111 (-86.069, 139.7067) -> (-85.6534, 139.7) centre (-85.6534, 152.654) ccw
  arc A112 (-99.7228, 108.5312) -> (-86.069, 139.7067) centre (-103.5908, 128.803) ccw
  arc A113 (-49.0754, 87.8375) -> (-30.5101, 92.7321) centre (-44.45, 107.95) ccw
  point P0 (0, 0)
  point P1 (-42.7408, 139.7)
  dimension "d105" = 6.35
  dimension "d106" = 6.35
  dimension "d107" = 6.35
  dimension "d108" = 3.175
  dimension "d109" = 3.175
  dimension "d110" = 6.35
  dimension "d111" = 3.175
  constraints: 104 point on circle, 94 end point, 45 centre point, 21 coincident, 21 point on line, 8 equal radius, 4 tangent, 1 collinear, 1 midpoint, 45 other
  measures "d105" distance between parallel lines of L0 L24
  measures "d106" radial gap between concentric circles of A1 A75
  measures "d107" radial gap between concentric circles of A48 A76
  measures "d108" distance between parallel lines of L38 L39
  measures "d109" distance between parallel lines of L37 L44
  measures "d110" distance between parallel lines of L14 L57
  measures "d111" distance between parallel lines of L63 L64
extrude "Extrusion5" cut sketch "Sketch7" against normal blind 25.4
fillet "Fillet3" radius 3.302 22 edges at (3.175, 78.3165, 19.8754) (3.175, 84.8824, 20.698) (3.175, 92.7321, 30.5101) (3.175, 87.8375, 49.0754) (3.175, 66.2974, 57.6915) (3.175, 59.2234, 55.242) (3.175, 54.2259, 46.586) (3.175, 55.4751, 38.7129) (3.175, 139.7, 42.7408) (3.175, 97.6906, 26.5433) (3.175, 89.841, 16.7312) (3.175, 87.9432, 6.35) (3.175, 134.3068, 6.35) (3.175, 139.7, 21.0312) (3.175, 139.7, 58.5025) (3.175, 139.7067, 86.069) (3.175, 108.5312, 99.7228) (3.175, 90.9051, 99.1218) (3.175, 68.2648, 81.075) (3.175, 65.3664, 70.1328) (3.175, 68.6557, 63.5873) (3.175, 90.1958, 54.9712)
body "Solid1"
